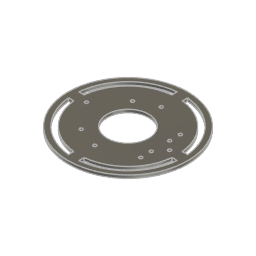
placa superior (Autodesk Fusion 360 design; units mm, degrees)
part number: 2026-06-22-13-42-12-689
Autodesk Fusion 360 part; units mm, degrees
note: some values were not read from the file. Set by a fixed rule: which sketch regions a step uses.
sketch "Boceto1" plane through (0, 0, 0) normal (0, 0, 1) x (1, 0, 0)
  circle A0 centre (0, 0) radius 57.5
  circle A1 centre (40, 0) radius 1.525
  circle A2 centre (-40, 0) radius 1.525
  circle A3 centre (0, -32) radius 1.525
  circle A4 centre (0, 32) radius 1.525
  dimension "d1" = 115
  dimension "d2" = 40
  dimension "d3" = 3.05
  dimension "d4" = 40
  dimension "d5" = 3.05
  dimension "d6" = 32
  dimension "d7" = 3.05
  dimension "d8" = 32
  dimension "d9" = 3.05
  constraint coincident A0.centre origin
  measures "d1" diameter of A0
  measures "d2" distance of A0.centre A1.centre
  measures "d3" diameter of A1
  measures "d4" distance of A0.centre A2.centre
  measures "d5" diameter of A2
  measures "d6" distance of A0.centre A3.centre
  measures "d7" diameter of A3
  measures "d8" distance of A0.centre A4.centre
  measures "d9" diameter of A4
extrude "Extruir1" add sketch "Boceto1" along normal blind 4
sketch "Boceto2" plane through (0, 0, 4) normal (0, 0, 1) x (-1, 0, 0)
  circle A0 centre (-40, 0) radius 1.525
  circle A1 centre (40, 0) radius 1.525
  circle A2 centre (0, -32) radius 1.525
  circle A3 centre (0, 32) radius 1.525
  circle A4 centre (0, 0) radius 57.5
  circle A5 centre (18.73, -23.1) radius 1.525
  circle A6 centre (-32.142, 19.9271) radius 1.525
  circle A7 centre (-32.142, -7.9554) radius 1.525
  circle A8 centre (-32.142, 9.758) radius 1.525
  circle A9 centre (-32.142, -18.182) radius 1.525
  circle A10 centre (20, 24.998) radius 1.525
  dimension "d19" = 3.05
  dimension "d20" = 3.05
  dimension "d21" = 3.05
  dimension "d32" = 27.94
  dimension "d33" = 3.05
  dimension "d35" = 3.05
  dimension "d43" = 3.05
  measures "d19" diameter of A5
  measures "d20" diameter of A6
  measures "d21" diameter of A7
  measures "d32" distance of A8.centre A9.centre
  measures "d33" diameter of A8
  measures "d35" diameter of A9
  measures "d43" diameter of A10
extrude "Extruir2" cut sketch "Boceto2" against normal blind 37 contours A5 | A6 | A7
extrude "Extruir3" cut 1 faces at (4.3667, -0.2928, 4) along direction (0, 0, -1) blind 1
sketch "Boceto3" plane through (0, 0, 3) normal (0, 0, 1) x (-1, 0, 0)
  circle A0 centre (0, 0) radius 57.5
  circle A1 centre (-40, 0) radius 1.525
  circle A2 centre (40, 0) radius 1.525
  circle A3 centre (0, 32) radius 1.525
  circle A4 centre (0, -32) radius 1.525
  circle A5 centre (18.73, -23.1) radius 1.525
  circle A6 centre (-32.142, 19.9271) radius 1.525
  circle A7 centre (-32.142, -7.9554) radius 1.525
  circle A8 centre (0, 0) radius 20
  dimension "d27" = 40
  constraint coincident A0.centre A8.centre
  measures "d27" diameter of A8
  measures "d43" diameter of A6.centre
extrude "Extruir4" cut sketch "Boceto3" against normal blind 5 contours A8
hole "Agujero1" at (32.142, -9.758, 4) at (32.142, 18.182, 4) direction (0, 0, -1) diameter 3 depth 10 tip angle 118
hole "Agujero2" at (-20, -24.998, 4) direction (0, 0, -1) diameter 3 depth 10 tip angle 118
sketch "Boceto4" plane through (0, 0, 3) normal (0, 0, 1) x (-1, 0, 0)
  circle A0 centre (-32.142, 9.758) radius 1.5
  circle A1 centre (-32.142, -18.182) radius 1.5
  circle A2 centre (-32.142, -7.9554) radius 1.525
  circle A3 centre (-32.142, 19.9271) radius 1.525
  circle A4 centre (18.73, -23.1) radius 1.525
  circle A5 centre (0, -32) radius 1.525
  circle A6 centre (0, 32) radius 1.525
  circle A7 centre (40, 0) radius 1.525
  circle A8 centre (-40, 0) radius 1.525
  circle A9 centre (0, 0) radius 57.5
  circle A10 centre (0, 0) radius 20
  circle A11 centre (20, 24.998) radius 1.5
  line L0 (5, -47.2361) -> (5, -52.2614)
  line L1 (-5, -47.2361) -> (-5, -52.2614)
  line L2 (5, 47.2361) -> (5, 52.2614)
  line L3 (-5, 47.2361) -> (-5, 52.2614)
  line L4 (52.2614, -5) -> (47.2361, -5)
  line L5 (-47.2361, -5) -> (-52.2614, -5)
  line L6 (52.2614, 5) -> (47.2361, 5)
  line L7 (-47.2361, 5) -> (-52.2614, 5)
  arc A12 (47.2361, 5) -> (5, 47.2361) centre (0, 0) ccw
  arc A13 (-5, 47.2361) -> (-47.2361, 5) centre (0, 0) ccw
  arc A14 (52.2614, 5) -> (5, 52.2614) centre (0, 0) ccw
  arc A15 (-5, 52.2614) -> (-52.2614, 5) centre (0, 0) ccw
  arc A16 (-47.2361, -5) -> (-5, -47.2361) centre (0, 0) ccw
  arc A17 (5, -47.2361) -> (47.2361, -5) centre (0, 0) ccw
  arc A18 (-52.2614, -5) -> (-5, -52.2614) centre (0, 0) ccw
  arc A19 (5, -52.2614) -> (52.2614, -5) centre (0, 0) ccw
  dimension "d47" = 105
  dimension "d48" = 95
  constraint concentric A9 A14
  constraint concentric A9 A12
  constraint coincident A9.centre A10.centre
  constraint collinear L4 L5
  constraint collinear L6 L7
  constraint concentric A12 A17
  constraint concentric A14 A19
  constraint concentric A12 A13
  constraint concentric A14 A15
  constraint concentric A16 A17
  constraint concentric A18 A19
  measures "d47" diameter of A14
  measures "d48" diameter of A12
extrude "Extruir5" cut sketch "Boceto4" against normal blind 5 contours L0 L4 A17 A19 | L1 L5 A16 A18 | L2 L6 A12 A14 | L3 L7 A13 A15
